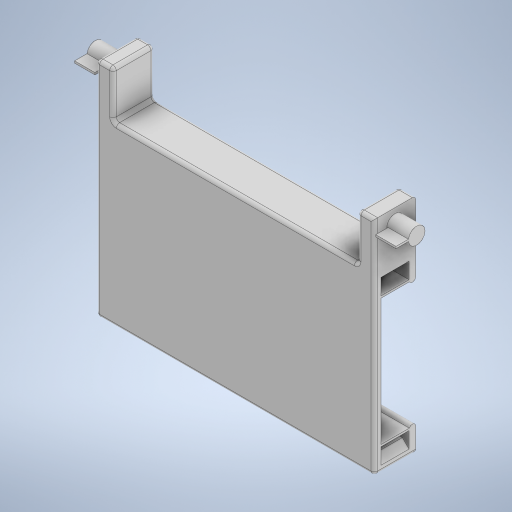
# Autodesk Inventor part: CaseV1
Saved by Autodesk Inventor 2024 (Build 280153000, 153)
## iProperties
Created: 2024-01-03
Part Number: CaseV1
Material: Generisch
Document SubType Name: Modeling
Designer: chris
Density: 1 g/cm^3
Appearance: Vorgabe
Author: chris
Autodesk Inventor part; units mm, degrees
ref_plane "YZ Plane" through (0, 0, 0) normal (1, 0, 0) x (0, 1, 0)
ref_plane "XZ Plane" through (0, 0, 0) normal (0, 1, 0) x (-1, 0, 0)
ref_plane "XY Plane" through (0, 0, 0) normal (0, 0, 1) x (1, 0, 0)
sketch "Skizze1" plane through (0, 0, 0) normal (0, 1, 0) x (-1, 0, 0)
  line L0 (-20.85, 11.2) -> (18.85, 11.2)
  line L1 (18.85, 11.2) -> (18.85, -11.2)
  line L2 (18.85, -11.2) -> (-20.85, -11.2)
  line L3 (-20.85, -11.2) -> (-20.85, 11.2)
  line L4 (-20.85, 11.2) -> (18.85, -11.2) construction
  line L5 (18.85, 11.2) -> (-20.85, -11.2) construction
  point P0 (0, 0)
  point P1 (-1, 0)
  dimension "d24" = 39.7
  dimension "d25" = 22.4
  dimension "d26" = 1
  dimension "d27" = 0
  constraints: 12 end point, 2 parallel, 1 horizontal, 1 midpoint, 1 perpendicular
  measures "d24" distance between parallel lines of L1 L3
  measures "d25" distance of L0.end L1.end
  measures "d26" distance of point (0, 0) point (-1, 0)
  measures "d27" vertical distance of point (0, 0) point (-1, 0)
extrude "Extrusion1" add sketch "Skizze1" along normal blind 1
sketch "Skizze2" plane through (0, 0, 0) normal (0, 1, 0) x (-1, 0, 0)
  line L0 (-20.85, 11.2) -> (-20.85, -11.2) projected
  line L1 (18.85, 11.2) -> (-20.85, 11.2) projected
  line L2 (20.85, -13.2) -> (-20.85, -13.2)
  line L3 (-20.85, -13.2) -> (-20.85, 13.2)
  line L4 (-20.85, 13.2) -> (20.85, 13.2)
  line L5 (20.85, 13.2) -> (20.85, -13.2)
  line L6 (20.85, -13.2) -> (-20.85, 13.2) construction
  line L7 (-20.85, -13.2) -> (20.85, 13.2) construction
  line L8 (18.85, -11.2) -> (18.85, 11.2) projected
  line L9 (-20.85, 11.2) -> (18.85, 11.2)
  line L10 (18.85, 11.2) -> (18.85, -11.2)
  line L11 (18.85, -11.2) -> (-20.85, -11.2)
  point P0 (0, 0)
  dimension "d30" = 2
  dimension "d31" = 2
  constraints: 18 end point, 3 perpendicular, 2 horizontal, 2 midpoint, 2 parallel
  measures "d30" distance between parallel lines of L1 L4
  measures "d31" distance between parallel lines of L8 L5
extrude "Extrusion2" add sketch "Skizze2" along normal blind 5.2 contours L3 L4 L5 L2 L11 L8 L1
sketch "Skizze3" plane through (0, 5.2, 0) normal (0, 1, 0) x (1, 0, 0)
  line L0 (20.85, 13.2) -> (-20.85, 13.2)
  line L1 (20.85, -13.2) -> (20.85, 13.2) projected
  line L2 (-20.85, 13.2) -> (20.85, 13.2)
  line L3 (20.85, 13.2) -> (20.85, -13.2)
  line L4 (20.85, -13.2) -> (-20.85, -13.2)
  line L5 (-20.85, -13.2) -> (-20.85, 13.2)
  line L6 (-20.85, 13.2) -> (20.85, -13.2) construction
  line L7 (20.85, 13.2) -> (-20.85, -13.2) construction
  line L8 (20.85, -11.2) -> (20.85, 11.2) projected
  line L9 (20.85, 9.2) -> (20.85, -9.2)
  line L10 (20.85, -11.2) -> (-18.85, -11.2) projected
  line L11 (-18.85, 11.2) -> (20.85, 11.2) projected
  line L12 (-18.85, -11.2) -> (-18.85, 11.2) projected
  line L13 (20.85, -9.2) -> (-18.85, -9.2)
  line L14 (-18.85, 9.2) -> (20.85, 9.2)
  point P0 (0, 0)
  point P1 (20.85, -9.2)
  dimension "d35" = 2
  dimension "d36" = 2
  constraints: 20 end point, 4 point on line, 3 perpendicular, 2 horizontal, 2 midpoint, 2 parallel
  measures "d35" distance between parallel lines of L10 L13
  measures "d36" distance between parallel lines of L11 L14
extrude "Extrusion3" add sketch "Skizze3" along normal blind 1 contours L1 L11 L12 L10 L4 L5 L0 | L1 L14 L12 L11 | L1 L10 L12 L13
sketch "Skizze7" plane through (20.85, 1, 11.2) normal (0, 0, -1) x (-1, 0, 0)
  line L0 (39.7, 4.2) -> (0, 4.2) construction
  line L1 (3.25, 4.2) -> (3.25, 0) construction
  line L2 (0, 0) -> (39.7, 0) construction
  line L3 (0, -1) -> (0, 5.2) construction
  circle A0 centre (3.25, 2.1) radius 0.75
  point P0 (20.85, -1)
  dimension "d38" = 1.5
  dimension "d39" = 2.5
  constraints: 2 end point, 2 point on line, 1 centre point, 1 midpoint, 1 vertical
  measures "d38" diameter of A0
  measures "d39" distance edge to line of A0 L3
extrude "Extrusion7" add sketch "Skizze7" along normal blind 0.3 draft -50
mirror "Spiegeln2" about plane through (0, 0, 0) normal (0, 0, 1) of "Extrusion7"
sketch "Skizze8" plane through (-20.85, 0, 13.2) normal (0, 0, 1) x (1, 0, 0)
  line L0 (0, 0) -> (0, 6.2) projected
  line L1 (41.7, 6.2) -> (2, 6.2) projected
  line L2 (0, 0) -> (2.5, 0)
  line L3 (2.5, 0) -> (2.5, 6.2)
  line L4 (2.5, 6.2) -> (0, 6.2)
  line L5 (0, 6.2) -> (0, 0)
  point P0 (20.85, 0)
  dimension "d42" = 2.5
  constraints: 8 end point, 2 parallel, 1 horizontal, 1 perpendicular, 1 point on line
  measures "d42" distance of L4.end L3.end
extrude "Extrusion8" add sketch "Skizze8" along normal blind 7
sketch "Skizze9" plane through (-20.85, 0, -13.2) normal (-1, 0, 0) x (0, 0, 1)
  line L0 (26.4, 6.2) -> (33.4, 6.2) construction
  line L1 (31.4, 6.2) -> (31.4, 0) construction
  line L2 (33.4, 6.2) -> (33.4, 0) construction
  circle A0 centre (31.4, 3.1) radius 1.25
  point P0 (13.2, 0)
  dimension "d45" = 2
  dimension "d46" = 2.5
  constraints: 2 end point, 1 centre point, 1 midpoint, 1 perpendicular, 1 point on line
  measures "d45" distance between parallel lines of L1 L2
  measures "d46" diameter of A0
extrude "Extrusion9" add sketch "Skizze9" along normal blind 3.25
mirror "Spiegeln3" about plane through (0, 0, 0) normal (1, 0, 0) of "Extrusion8", "Extrusion9"
sketch "Skizze11" plane through (0, 1, 0) normal (0, 1, 0) x (1, 0, 0)
  line L0 (20.85, -11.2) -> (20.85, 11.2) projected
  line L1 (20.85, -9.5) -> (-18.45, -9.5)
  line L2 (-18.45, -9.5) -> (-18.45, -9.8)
  line L3 (-18.45, -9.8) -> (20.85, -9.8)
  line L4 (20.85, -9.8) -> (20.85, -9.5)
  line L5 (-18.85, -11.2) -> (-18.85, -9.2) projected
  line L6 (20.85, -9.2) -> (-18.85, -9.2) projected
  point P0 (0, 0)
  point P1 (-18.45, -9.65)
  dimension "d50" = 0.3
  dimension "d51" = 0.4
  dimension "d54" = 0.3
  constraints: 8 end point, 2 parallel, 1 horizontal, 1 midpoint, 1 perpendicular, 1 point on line
  measures "d50" distance between parallel lines of L3 L1
  measures "d51" distance from line of point (-18.45, -9.65) L5
  measures "d54" distance between parallel lines of L1 L6
extrude "Extrusion10" add sketch "Skizze11" along normal up to surface (4.2 mm away)
mirror "Spiegeln4" about plane through (0, 0, 0) normal (0, 0, 1) of "Extrusion10"
sketch "Skizze12" plane through (0, 0, 0) normal (0, 1, 0) x (-1, 0, 0)
  line L0 (-20.85, 9.2) -> (-20.85, 20.2) construction
  line L1 (-24.1, 18.35) -> (-21.05, 18.35)
  line L2 (-21.05, 18.35) -> (-21.05, 18.05)
  line L3 (-21.05, 18.05) -> (-24.1, 18.05)
  line L4 (-24.1, 16.95) -> (-24.1, 19.45) construction
  line L5 (-24.1, 18.2) -> (-20.85, 18.2) construction
  line L6 (-24.1, 18.35) -> (-24.1, 18.05)
  point P0 (0, 0)
  dimension "d55" = 0.15
  dimension "d56" = 0.15
  dimension "d57" = 0.2
  constraints: 10 end point, 2 perpendicular, 1 horizontal, 1 midpoint, 1 point on line
  measures "d55" distance between parallel lines of L1 L5
  measures "d56" distance between parallel lines of L3 L5
  measures "d57" distance between parallel lines of L0 L2
extrude "Extrusion11" add sketch "Skizze12" along normal up to surface round surface about axis through (20.85, 3.1, 18.2) along (-1, 0, 0) radius 1.25 far side no
mirror "Spiegeln5" about plane through (0, 0, 0) normal (1, 0, 0) of "Extrusion11"
fillet "Rundung1" radius 0.5 4 edges at (1, 6.2, -9.2) (1, 5.2, -9.2) (1, 6.2, 9.2) (1, 5.2, 9.2)
fillet "Rundung2" radius 0.5 4 edges at (0, 6.2, -13.2) (20.85, 3.1, -13.2) (0, 0, -13.2) (-20.85, 3.1, -13.2)
fillet "Rundung3" radius 0.5 10 edges at (0, 0, 13.2) (0, 6.2, 13.2) (18.35, 3.1, 13.2) (-18.35, 3.1, 13.2) (-18.35, 6.2, 16.7) (-18.35, 0, 16.7) (-18.35, 3.1, 20.2) (18.35, 6.2, 16.7) (18.35, 3.1, 20.2) (18.35, 0, 16.7)
fillet "Rundung4" radius 0.5 14 edges at (20.7036, 0.1464, -13.0536) (20.85, 0, 3.75) (-20.7036, 0.1464, -13.0536) (-20.85, 0, 3.75) (-20.7036, 6.0536, -13.0536) (-20.85, 6.2, 3.75) (18.4964, 6.0536, 20.0536) (19.85, 6.2, 20.2) (18.4964, 0.1464, 20.0536) (19.85, 0, 20.2) (-18.4964, 6.0536, 20.0536) (-19.85, 6.2, 20.2) (-18.4964, 0.1464, 20.0536) (-19.85, 0, 20.2)
chamfer "Fasen1" distance 1 angle 45 2 edges at (20.85, 3.1, 11.2) (20.85, 3.1, -11.2)
fillet "Rundung5" radius 0.5 3 edges at (-20.7036, 0.1464, 20.0536) (-20.7036, 6.0536, 20.0536) (-20.85, 3.1, 20.2)
fillet "Rundung6" radius 0.25 1 edges at (-18.85, 6.2, 0)
